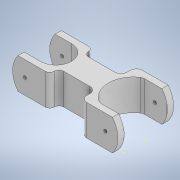
# Autodesk Inventor part: PartArm
Saved by Autodesk Inventor 2022 (Build 260153000, 153)
## iProperties
Created: 2022-01-07
Part Number: PartArm
Material: Generic
Document SubType Name: Modeling
Designer: nguye
Density: 1 g/cm^3
Appearance: Default
Author: nguye
Autodesk Inventor part; units mm, degrees
ref_plane "YZ Plane" through (0, 0, 0) normal (1, 0, 0) x (0, 1, 0)
ref_plane "XZ Plane" through (0, 0, 0) normal (0, 1, 0) x (-1, 0, 0)
ref_plane "XY Plane" through (0, 0, 0) normal (0, 0, 1) x (1, 0, 0)
sketch "Sketch1" plane through (0, 0, 0) normal (0, 1, 0) x (-1, 0, 0)
  line L0 (100, -45) -> (0, -45)
  line L1 (0, -45) -> (0, 0)
  line L2 (100, 45) -> (0, 45)
  line L3 (0, 45) -> (0, 0)
  line L4 (100, -45) -> (180, -45)
  line L5 (100, 45) -> (180, 45)
  line L6 (180, -45) -> (180, 45)
  dimension "d0" = 100
  constraints: 14 end point, 1 perpendicular
  measures "d0" distance of L0.start L0.end
extrude "Extrusion1" add sketch "Sketch1" along normal blind 50
sketch "Sketch2" plane through (0, 50, 0) normal (0, 1, 0) x (1, 0, 0)
  line L0 (-180, -45) -> (0, -45) projected
  line L1 (-60, -45) -> (-60, 45)
  line L2 (0, 45) -> (-180, 45) projected
  line L3 (-120, 45) -> (-120, -45)
  line L4 (-60, 0) -> (-60, 20)
  line L5 (-60, 20) -> (-60, 0)
  line L6 (-60, 0) -> (-60, -20)
  line L7 (-60, -20) -> (-120, -20)
  line L8 (-60, 20) -> (-120, 20)
  line L9 (-180, -45) -> (0, -45)
  line L10 (0, 45) -> (-180, 45)
  line L11 (-180, 45) -> (-180, -45) projected
  line L12 (-180, -45) -> (-180, 45)
  line L13 (-180, -25) -> (-180, -15)
  line L14 (-180, 25) -> (-180, 15)
  line L15 (0, -45) -> (0, 45) projected
  line L16 (0, 45) -> (0, 35)
  line L17 (0, 35) -> (-60, 35)
  line L18 (0, -45) -> (0, -35)
  line L19 (0, -35) -> (-60, -35)
  line L20 (0, 0) -> (-20, 0)
  arc A0 (-0.6351, -35) -> (0, -34.641) centre (-20, 0) ccw
  arc A1 (0, 34.641) -> (-0.6351, 35) centre (-20, 0) ccw
  arc A2 (-39.3649, 35) -> (-39.3649, -35) centre (-20, 0) ccw
  line L21 (-120, 35) -> (-180, 35)
  line L22 (-120, -35) -> (-180, -35)
  line L23 (-180, 35) -> (-180, 25)
  line L24 (-180, 25) -> (-145, 25)
  line L25 (-180, -35) -> (-180, -25)
  line L26 (-180, -25) -> (-145, -25)
  arc A3 (-145, -25) -> (-145, 25) centre (-145, 0) ccw
  dimension "d5" = 60
  dimension "d13" = 20
  dimension "d14" = 20
  dimension "d18" = 10
  dimension "d19" = 10
  dimension "d25" = 10
  dimension "d26" = 10
  dimension "d27" = 20
  dimension "d28" = 10
  dimension "d29" = 10
  constraints: 46 end point, 22 point on line, 9 point on circle, 8 perpendicular, 4 centre point, 4 collinear, 2 horizontal, 1 coincident, 1 parallel
  measures "d5" distance of L0.end L1.start
  measures "d13" distance of L4.start L4.end
  measures "d14" distance of L4.start L6.end
  measures "d18" distance of L13.start L13.end
  measures "d19" distance of L14.start L14.end
  measures "d25" distance of L2.start L16.end
  measures "d26" distance of L0.end L18.end
  measures "d27" distance of L20.start L20.end
  measures "d28" distance of L21.end L14.start
  measures "d29" distance of L22.end L13.start
extrude "Extrusion2" cut sketch "Sketch2" against normal blind 50 contours L11 L22 L3 L0 | L3 L7 L1 L0 | L11 L24 A3 L26 | A2 L17 A1 L15 A0 L19 | L3 L2 L1 L8 | L21 L11 L2 L3
fillet "Fillet1" radius 10 1 edges at (-39.3649, 25, 35)
fillet "Fillet2" radius 10 1 edges at (-39.3649, 25, -35)
fillet "Fillet3" radius 10 1 edges at (-60, 25, 45)
fillet "Fillet4" radius 10 3 edges at (-60, 25, 20) (-60, 25, -20) (-60, 25, -45)
fillet "Fillet5" radius 7.5 1 edges at (-120, 25, 35)
fillet "Fillet6" radius 7.5 3 edges at (-120, 25, 20) (-120, 25, -20) (-120, 25, -35)
sketch "Sketch3" plane through (-180, 0, -35) normal (0, 0, -1) x (-1, 0, 0)
  line L0 (0, 0) -> (0, 50) projected
  arc A0 (-8.775, 0) -> (-8.775, 50) centre (-40, 25) ccw
  line L1 (0, 50) -> (-52.5, 50) projected
  line L2 (0, 50) -> (-8.775, 50)
  line L3 (-8.775, 0) -> (0, 0)
  line L4 (0, 0) -> (0, 50)
  line L5 (-180, 0) -> (-180, 50) projected
  arc A1 (-171.225, 50) -> (-171.225, 0) centre (-140, 25) ccw
  line L6 (-130, 0) -> (-180, 0) projected
  line L7 (-180, 0) -> (-171.225, 0)
  line L8 (-171.225, 50) -> (-180, 50)
  line L9 (-180, 50) -> (-180, 0)
  point P0 (-180, 25)
  point P1 (-171.225, 0)
  point P2 (-8.775, 50)
  point P3 (0, 25)
  constraints: 12 end point, 4 point on circle, 2 centre point, 2 horizontal, 2 parallel
extrude "Extrusion3" cut sketch "Sketch3" along normal mid plane 200
sketch "Sketch4" plane through (-50, 0, -45) normal (0, 0, -1) x (-1, 0, 0)
  arc A0 (-41.225, 50) -> (-41.225, 0) centre (-10, 25) ccw projected
  circle A1 centre (-30, 25) radius 2.5
  arc A2 (121.225, 0) -> (121.225, 50) centre (90, 25) ccw projected
  circle A3 centre (110, 25) radius 2.5
  point P0 (-50, 0)
  dimension "d44" = 5
  dimension "d46" = 5
  constraints: 2 centre point
  measures "d44" diameter of A1
  measures "d46" diameter of A3
extrude "Extrusion4" cut sketch "Sketch4" against normal blind 200
sketch "Sketch5" plane through (0, 0, 0) normal (0, -1, 0) x (1, 0, 0)
  point P0 (0, 0)
sketch "Sketch6" plane through (-127.5, 0, 35) normal (0, 0, 1) x (1, 0, 0)
  point P0 (127.5, 0)
body "Solid1"
